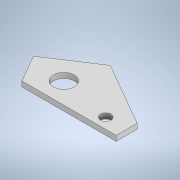
# Autodesk Inventor part: SliderBlock
Saved by Autodesk Inventor 2022.2 (Build 262287030, 287C)
## iProperties
Created: 2023-02-08
Part Number: SliderBlock
Material: Generic
Document SubType Name: Modeling
Designer: jak27277
Density: 1 g/cm^3
Appearance: Default
Author: jak27277
Autodesk Inventor part; units mm, degrees
ref_plane "YZ Plane" through (0, 0, 0) normal (1, 0, 0) x (0, 1, 0)
ref_plane "XZ Plane" through (0, 0, 0) normal (0, 1, 0) x (-1, 0, 0)
ref_plane "XY Plane" through (0, 0, 0) normal (0, 0, 1) x (1, 0, 0)
sketch "Sketch1" plane through (0, 0, 0) normal (0, 1, 0) x (-1, 0, 0)
  circle A0 centre (0, 0) radius 12.7
  line L0 (-11.9103, -44.45) -> (44.45, -7.5956)
  line L1 (44.45, -7.5956) -> (25.4, 25.4)
  line L2 (25.4, 25.4) -> (-88.9, 25.4)
  line L3 (-88.9, 25.4) -> (-88.9, 0)
  line L4 (-88.9, 0) -> (-11.9103, -44.45)
  circle A1 centre (-63.5, 12.7) radius 6.35
  dimension "d0" = 60
  dimension "d1" = 60
  dimension "d2" = 25.4
  dimension "d3" = 25.4
  dimension "d4" = 25.4
  dimension "d5" = 88.9
  dimension "d6" = 88.9
  dimension "d7" = 114.3
  dimension "d8" = 12.7
  dimension "d9" = 25.4
  dimension "d10" = 12.7
  dimension "d11" = 38.1
  constraints: 10 end point, 2 centre point, 1 coincident, 1 horizontal, 1 perpendicular
  measures "d0" angle of L2 L1
  measures "d1" angle of L4 L3
  measures "d2" distance from line of L2 point (0, 0)
  measures "d3" diameter of A0
  measures "d4" distance of L2.end L3.end
  measures "d5" distance of L3.end L0.start
  measures "d6" distance from line of L3 point (0, 0)
  measures "d7" distance of L1.end L2.end
  measures "d8" diameter of A1
  measures "d9" distance from line of L3 A1.centre
  measures "d10" distance from line of L2 A1.centre
  measures "d11" distance of L0.end L1.end
extrude "Extrusion1" add sketch "Sketch1" along normal blind 6.35
body "Solid1"
